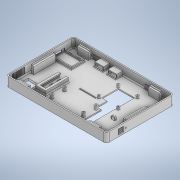
# Autodesk Inventor part: Bottom_new
Saved by Autodesk Inventor 2021 (Build 250183000, 183)
## iProperties
Created: 2020-06-14
Part Number: Bottom_new
Material: Generic
Document SubType Name: Modeling
Designer: Mariano
Density: 1 g/cm^3
Appearance: Default
Author: Mariano
Autodesk Inventor part; units mm, degrees
(part 1 of 3)
ref_plane "YZ Plane" through (0, 0, 0) normal (1, 0, 0) x (0, 1, 0)
ref_plane "XZ Plane" through (0, 0, 0) normal (0, 1, 0) x (-1, 0, 0)
sketch "Sketch1" plane through (0, 0, 0) normal (0, 1, 0) x (-1, 0, 0)
  line L0 (92.2, -62) -> (-92.2, -62)
  line L1 (-92.2, -62) -> (-92.2, 62)
  line L2 (-92.2, 62) -> (92.2, 62)
  line L3 (92.2, 62) -> (92.2, -62)
  line L4 (92.2, -62) -> (-92.2, 62) construction
  line L5 (-92.2, -62) -> (92.2, 62) construction
  point P0 (0, 0)
  dimension "d0" = 184.4
  dimension "d1" = 124
  constraints: 12 end point, 2 midpoint, 2 parallel, 1 horizontal, 1 perpendicular
  measures "d0" distance of L1.end L2.end
  measures "d1" distance of L2.end L0.start
extrude "Extrusion1" add sketch "Sketch1" along normal blind 17
fillet "Fillet1" radius 5 4 edges at (-92.2, 8.5, 62) (92.2, 8.5, 62) (92.2, 8.5, -62) (-92.2, 8.5, -62)
shell "Shell1" thickness 2 removed faces 1 at (29.0667, 17, 20.6667)
ref_plane "Work Plane4" through (0, 0, 20) normal (0, 0, 1) x (1, 0, 0)
sketch "Sketch28" plane through (0, 0, 20) normal (0, 0, 1) x (1, 0, 0)
  circle A0 centre (62.2, 4.5) radius 4
  line L0 (92.2, 17) -> (92.2, 0) projected
  circle A1 centre (62.2, 4.5) radius 2.5
  line L1 (58.2, 4.5) -> (58.2, 2)
  line L2 (87.2, 2) -> (-87.2, 2) construction
  line L3 (60.1894, 5.9858) -> (60.1894, 7.958)
  line L4 (64.2106, 5.9858) -> (64.2106, 7.958)
  line L5 (66.2, 4.5) -> (66.2, 2)
  point P0 (0, 0)
  point P1 (75.2, 2)
  dimension "d152" = 8
  dimension "d153" = 30
  dimension "d156" = 5
  dimension "d157" = 4.0211
  dimension "d158" = 1.9722
  constraints: 8 end point, 6 point on circle, 3 tangent, 2 centre point, 2 vertical, 1 coincident, 1 parallel, 1 perpendicular, 1 point on line
  measures "d152" diameter of A0
  measures "d153" distance from line of L0 A0.centre
  measures "d156" diameter of A1
  measures "d157" distance of L4.start L3.start
  measures "d158" distance of L4.start L4.end
extrude "Extrusion21" add sketch "Sketch28" against normal blind 3 contours A0 L3 A1 L4 picked at (65.6381, 3.986)
fillet "Fillet3" radius 10.5 2 edges at (60.1894, 5.9858, 18.5) (64.2106, 5.9858, 18.5)
ref_plane "Work Plane5" through (0, 16, 0) normal (0, 1, 0) x (1, 0, 0)
sketch "Sketch31" plane through (-87.2, 2, 60) normal (0, 1, 0) x (1, 0, 0)
  line L0 (2, 114.9) -> (172.4, 114.9) construction
  line L1 (172.4, 114.9) -> (172.4, 3) construction
  line L2 (172.4, 3) -> (2, 3) construction
  line L3 (2, 3) -> (2, 114.9) construction
  line L4 (87.2, 114.9) -> (87.2, 3) construction
  line L5 (2, 58.95) -> (172.4, 58.95) construction
  line L6 (12, 116.9) -> (32, 116.9)
  line L7 (32, 116.9) -> (32, 111.9)
  line L8 (32, 111.9) -> (12, 111.9)
  line L9 (12, 111.9) -> (12, 116.9)
  line L10 (0, 78.95) -> (5, 78.95)
  line L11 (5, 78.95) -> (5, 38.95)
  line L12 (4, 38.95) -> (0, 38.95)
  line L13 (0, 38.95) -> (0, 78.95)
  line L14 (174.4, 0) -> (0, 0) projected
  line L15 (0, 38.95) -> (5, 38.95)
  point P0 (87.2, 60)
  point P1 (32, 114.4)
  point P2 (5, 58.95)
  point P3 (2, 38.95)
  point P4 (4, 38.95)
  dimension "d188" = 170.4
  dimension "d189" = 111.9
  dimension "d190" = 20
  dimension "d191" = 5
  dimension "d192" = 10
  dimension "d198" = 40
  dimension "d199" = 5
  dimension "d256" = 3
  dimension "d389" = 3
  dimension "d502" = 2
  constraints: 30 end point, 7 midpoint, 7 parallel, 3 horizontal, 3 perpendicular, 3 point on line, 1 collinear
  measures "d188" distance of L0.start L0.end
  measures "d189" distance of L0.end L1.end
  measures "d190" distance of L7.end L8.end
  measures "d191" distance of L6.end L7.end
  measures "d192" distance between parallel lines of L3 L9
  measures "d198" distance of L10.end L11.end
  measures "d199" distance between parallel lines of L11 L13
  measures "d256" distance between parallel lines of L14 L2
  measures "d389" distance between parallel lines of L8 L0
  measures "d502" distance between parallel lines of L13 L3
extrude "Extrusion22" add sketch "Sketch31" along normal up to surface (14 mm away) contours L6 L7 L8 L9
sketch "Sketch32" plane through (-75.2, 16, -51.9) normal (0, 1, 0) x (1, 0, 0)
  line L0 (0, 0) -> (0, 6)
  line L1 (0, 3) -> (20, 3)
  line L2 (20, 6) -> (20, 0)
  line L3 (20, 0) -> (0, 0) projected
  line L4 (20, 0) -> (0, 0)
  line L5 (0, 0) -> (0, 3)
  point P0 (75.2, -51.9)
  dimension "d390" = 3
  constraints: 10 end point, 2 midpoint, 1 collinear, 1 perpendicular
  measures "d390" distance between parallel lines of L1 L3
extrude "Extrusion23" cut sketch "Sketch32" against normal blind 1.2
extrude "Extrusion24" add sketch "Sketch31" along normal up to surface (14 mm away) contours L10 L11 L15 L12 L13
sketch "Sketch33" plane through (-87.2, 16, 21.05) normal (0, 1, 0) x (1, 0, 0)
  line L0 (5, 40) -> (5, 0) projected
  line L1 (1.8, 0) -> (5, 0)
  line L2 (5, 0) -> (5, 40)
  line L3 (5, 40) -> (1.8, 40)
  line L4 (1.8, 40) -> (1.8, 0)
  line L5 (0, 0) -> (0, 40) projected
  point P0 (87.2, 21.05)
  dimension "d503" = 1.8
  constraints: 8 end point, 2 parallel, 1 horizontal, 1 perpendicular
  measures "d503" distance between parallel lines of L4 L5
extrude "Extrusion25" cut sketch "Sketch33" against normal blind 1.2
mirror "Mirror13" about plane through (0, 0, 0) normal (1, 0, 0) of "Extrusion24", "Extrusion25"
sketch "Sketch34" plane through (-87.2, 2, 60) normal (0, 1, 0) x (1, 0, 0)
  line L0 (103.971, 95) -> (134.4, 95)
  line L1 (134.4, 95) -> (134.4, 64.596)
  line L2 (134.4, 64.596) -> (103.971, 64.596)
  line L3 (103.971, 64.596) -> (103.971, 95)
  circle A0 centre (101.469, 97.502) radius 2.502
  line L4 (119.1855, 95) -> (119.1855, 64.596) construction
  line L5 (103.971, 79.798) -> (134.4, 79.798) construction
  circle A1 centre (136.902, 97.502) radius 2.502
  circle A2 centre (101.469, 62.094) radius 2.502
  circle A3 centre (136.902, 62.094) radius 2.502
  line L6 (0, 120) -> (174.4, 120) projected
  line L7 (177.4, 117) -> (177.4, 3) projected
  line L8 (109.4, 64.596) -> (134.4, 64.596)
  line L9 (134.4, 64.596) -> (134.4, 4.596)
  line L10 (134.4, 4.596) -> (122.4, 4.596)
  line L11 (122.4, 4.596) -> (122.4, 45.596)
  line L12 (122.4, 45.596) -> (114, 45.596)
  line L13 (114, 45.596) -> (114, 64.596)
  point P0 (87.2, 60)
  dimension "d204" = 30.429
  dimension "d205" = 30.404
  dimension "d206" = 5.004
  dimension "d207" = 2.502
  dimension "d208" = 2.502
  dimension "d209" = 25
  dimension "d210" = 43
  dimension "d227" = 12
  dimension "d228" = 60
  dimension "d387" = 20.4
  dimension "d388" = 41
  constraints: 24 end point, 4 centre point, 4 midpoint, 4 perpendicular, 3 parallel, 3 point on line, 3 symmetric about line, 2 horizontal, 1 vertical, 3 other
  measures "d204" distance of L1.end L2.end
  measures "d205" distance of L0.end L1.end
  measures "d206" diameter of A0
  measures "d207" distance from line of L3 A0.centre
  measures "d208" distance from line of L0 A0.centre
  measures "d209" distance between parallel lines of L0 L6
  measures "d210" distance between parallel lines of L7 L1
  measures "d227" distance of L9.end L10.end
  measures "d228" distance between parallel lines of L10 L2
  measures "d387" distance between parallel lines of L9 L13
  measures "d388" distance of L10.end L11.end
extrude "Extrusion27" add sketch "Sketch34" along normal blind 4 contours A3 | A0 | A1 | A2
extrude "Extrusion28" cut sketch "Sketch34" against normal through all contours L0 L1 L2 L3
extrude "Extrusion29" cut sketch "Sketch34" against normal through all contours L0 L1 L2 L3 | L9 L10 L11 L12 L13 L2
sketch "Sketch36" plane through (-87.2, 2, 60) normal (0, 1, 0) x (1, 0, 0)
  line L0 (22.24, 13) -> (7, 13)
  line L1 (7, 13) -> (7, 26.5)
  line L2 (7, 26.5) -> (22.24, 26.5)
  line L3 (22.24, 26.5) -> (22.24, 13)
  circle A0 centre (19.7, 11.26) radius 1.275
  line L4 (14.62, 13) -> (14.62, 26.5) construction
  circle A1 centre (9.54, 11.26) radius 1.275
  line L5 (0, 120) -> (174.4, 120) projected
  line L6 (-3, 3) -> (-3, 117) projected
  line L7 (-5, 117) -> (-5, 3) projected
  line L8 (0, -2) -> (174.4, -2) projected
  point P0 (87.2, 60)
  dimension "d231" = 15.24
  dimension "d232" = 13.5
  dimension "d233" = 2.55
  dimension "d234" = 15.24
  dimension "d235" = 2.54
  dimension "d511" = 12
  dimension "d512" = 15
  constraints: 10 end point, 2 centre point, 2 midpoint, 2 parallel, 1 perpendicular, 1 symmetric about line, 1 other
  measures "d231" distance of L1.end L2.end
  measures "d232" distance of L0.end L1.end
  measures "d233" diameter of A0
  measures "d234" distance from line of L2 A0.centre
  measures "d235" distance from line of L3 A0.centre
  measures "d511" distance between parallel lines of L7 L1
  measures "d512" distance between parallel lines of L8 L0
extrude "Extrusion30" add sketch "Sketch36" along normal blind 4 contours A0 | A1
extrude "Extrusion31" cut sketch "Sketch36" against normal through all contours L0 L1 L2 L3
sketch "Sketch35" plane through (-87.2, 2, 60) normal (0, 1, 0) x (1, 0, 0)
  line L0 (54.7, 45.5337) -> (119.7, 45.5337) construction
  line L1 (119.7, 45.5337) -> (119.7, 15.3337) construction
  line L2 (119.7, 15.3337) -> (54.7, 15.3337) construction
  line L3 (54.7, 15.3337) -> (54.7, 45.5337) construction
  circle A0 centre (58.2, 42.0337) radius 3
  line L4 (87.2, 45.5337) -> (87.2, 15.3337) construction
  line L5 (54.7, 30.4337) -> (119.7, 30.4337) construction
  circle A1 centre (116.2, 42.0337) radius 3
  circle A2 centre (58.2, 19.0337) radius 3
  line L6 (54.7, 15.3337) -> (119.7, 15.3337) construction
  circle A3 centre (116.2, 19.0337) radius 3
  point P0 (87.2, 60)
  dimension "d211" = 65
  dimension "d212" = 30.2
  dimension "d213" = 6
  dimension "d214" = 3.5
  dimension "d215" = 3.5
  dimension "d216" = 6
  dimension "d217" = 3.5
  dimension "d218" = 3.7
  constraints: 14 end point, 4 centre point, 4 midpoint, 4 symmetric about line, 2 parallel, 1 horizontal, 1 perpendicular, 1 point on line, 2 other
  measures "d211" distance of L1.end L2.end
  measures "d212" distance of L0.end L1.end
  measures "d213" diameter of A0
  measures "d214" distance from line of L0 A0.centre
  measures "d215" distance from line of L3 A0.centre
  measures "d216" diameter of A2
  measures "d217" distance from line of L3 A2.centre
  measures "d218" distance from line of L2 A2.centre
extrude "Extrusion26" add sketch "Sketch35" along normal blind 6
sketch "Sketch37" plane through (-29, 8, 40.9663) normal (0, 1, 0) x (1, 0, 0)
  circle A0 centre (0, 0) radius 3 projected
  circle A1 centre (0, 23) radius 3 projected
  circle A2 centre (58, 0) radius 3 projected
  circle A3 centre (58, 23) radius 3 projected
  point P0 (29, 40.9663)
  point P1 (0, 23)
  point P2 (58, 0)
  point P3 (58, 23)
  constraints: 4 coincident
hole "Hole10" at (-29, 8, 40.9663) at (-29, 8, 17.9663) at (29, 8, 40.9663) at (29, 8, 17.9663) direction (0, -1, 0) diameter 3 depth 6 tip angle 118
sketch "Sketch38" plane through (14.269, 6, -2.094) normal (0, 1, 0) x (1, 0, 0)
  circle A0 centre (0, 0) radius 2.502 projected
  circle A1 centre (0, 35.408) radius 2.502 projected
  circle A2 centre (35.433, 0) radius 2.502 projected
  arc A3 (37.935, 35.408) -> (37.935, 35.408) centre (35.433, 35.408) ccw projected
  point P0 (-14.269, -2.094)
  point P1 (0, 35.408)
  point P2 (35.433, 0)
  point P3 (35.433, 35.408)
  constraints: 4 coincident
hole "Hole11" at (14.269, 6, -2.094) at (14.269, 6, -37.502) at (49.702, 6, -2.094) at (49.702, 6, -37.502) direction (0, -1, 0) diameter 2 depth 4 tip angle 118
ref_plane "Work Plane8" through (-85.2, 2, 1.05) normal (0, 0, 1) x (1, 0, 0)
ref_plane "Work Plane9" through (0, 2, -54.9) normal (-1, 0, 0) x (0, 0, 1)
mirror "Mirror14" about plane through (0, 2, -54.9) normal (-1, 0, 0) of "Extrusion22", "Extrusion23"
mirror "Mirror15" about plane through (-85.2, 2, 1.05) normal (0, 0, 1) of "Extrusion22", "Extrusion23", "Mirror14"
sketch "Sketch40" plane through (-87.2, 2, -60) normal (0, 0, 1) x (1, 0, 0)
  line L0 (34, 7) -> (46, 7)
  line L1 (46, 7) -> (46, 5)
  line L2 (46, 5) -> (34, 5)
  line L3 (34, 5) -> (34, 7)
  line L4 (-5, 15) -> (0, 15) projected
  line L5 (0, 15) -> (0, -2) projected
  line L6 (0, -2) -> (-5, -2) projected
  line L7 (-5, -2) -> (-5, 15) projected
  line L8 (0, 15) -> (174.4, 15) projected
  point P0 (87.2, -2)
  dimension "d260" = 2
  dimension "d261" = 12
  dimension "d262" = 39
  dimension "d510" = 8
  constraints: 8 end point, 2 parallel, 1 horizontal, 1 perpendicular
  measures "d260" distance of L2.end L0.start
  measures "d261" distance of L1.end L2.end
  measures "d262" distance between parallel lines of L7 L3
  measures "d510" distance between parallel lines of L8 L0
extrude "Extrusion32" cut sketch "Sketch40" against normal blind 1.2 contours L0 L1 L2 L3
mirror "Mirror16" about plane through (0, 0, 0) normal (1, 0, 0) of "Extrusion32"
mirror "Mirror17" about plane through (0, 0, 0) normal (0, 0, 1) of "Extrusion32", "Mirror16"
sketch "Sketch44" plane through (-90.2, 2, -57) normal (1, 0, 0) x (0, 0, -1)
  line L0 (-63, 7) -> (-51, 7)
  line L1 (-51, 7) -> (-51, 5)
  line L2 (-51, 5) -> (-63, 5)
  line L3 (-63, 5) -> (-63, 7)
  line L4 (0, 15) -> (0, 0) projected
  line L5 (-114, 15) -> (0, 15) projected
  line L6 (-118, 15) -> (-114, 15) projected
  line L7 (-118, -2) -> (-118, 15) projected
  line L8 (4, -2) -> (-118, -2) projected
  line L9 (4, 15) -> (4, -2) projected
  line L10 (0, 15) -> (4, 15) projected
  line L11 (-114, 0) -> (0, 0) projected
  line L12 (-114, 15) -> (-114, 0) projected
  line L13 (0, 15) -> (0, 0) projected
  line L14 (-118, -2) -> (-118, 15) projected
  line L15 (4, -2) -> (-118, -2) projected
  line L16 (4, 15) -> (4, -2) projected
  line L17 (-114, 0) -> (0, 0) projected
  line L18 (-114, 15) -> (-114, 0) projected
  line L19 (-114, 15) -> (-119, 15) projected
  line L20 (-119, 15) -> (-119, -2) projected
  line L21 (-119, -2) -> (-114, -2) projected
  line L22 (-114, -2) -> (-114, 15) projected
  line L23 (-114, 0) -> (0, 0) projected
  line L24 (0, 15) -> (0, 0) projected
  line L25 (-118, -2) -> (-118, 15) projected
  line L26 (4, -2) -> (-118, -2) projected
  line L27 (4, 15) -> (4, -2) projected
  line L28 (-114, 15) -> (-114, 0) projected
  line L29 (29.8, -2) -> (-143.8, -2) projected
  line L30 (-57, -5.4) -> (-57, 18.4) projected
  line L31 (-114, 15) -> (0, 15) projected
  line L32 (-118, 15) -> (-114, 15) projected
  line L33 (0, 15) -> (4, 15) projected
  line L34 (-114, 15) -> (0, 15) projected
  line L35 (-118, 15) -> (-114, 15) projected
  line L36 (0, 15) -> (4, 15) projected
  point P0 (-57, -2)
  point P1 (-57, 5)
  dimension "d266" = 12
  dimension "d267" = 2
  dimension "d508" = 8
  constraints: 8 end point, 2 parallel, 1 horizontal, 1 midpoint, 1 perpendicular, 1 point on line
  measures "d266" distance of L1.end L2.end
  measures "d267" distance of L0.end L1.end
  measures "d508" distance between parallel lines of L5 L0
extrude "Extrusion33" cut sketch "Sketch44" against normal blind 1.2 contours L0 L30 L2 L3 | L0 L1 L2 L30
chamfer "Chamfer6" distance 2 angle 45 8 edges at (-90.2, 2, 0) (-89.3213, 2, -59.1213) (0, 2, -60) (89.3213, 2, -59.1213) (90.2, 2, 0) (-89.3213, 2, 59.1213) (0, 2, 60) (89.3213, 2, 59.1213)
ref_plane "Work Plane10" through (-87.2, 15.4, 21.05) normal (0, 1, 0) x (1, 0, 0)
sketch "Sketch50" plane through (-87.2, 15.4, 21.05) normal (0, 1, 0) x (1, 0, 0)
  line L0 (-3, 78.05) -> (-3, -35.95) projected
  line L1 (-1, -35.95) -> (-1, 78.05) projected
  line L2 (-3, 15.05) -> (-1, 15.05)
  line L3 (-1, 15.05) -> (-1, 27.05)
  line L4 (-1, 27.05) -> (-3, 27.05)
  line L5 (-3, 27.05) -> (-3, 15.05)
  point P0 (87.2, 21.05)
  point P1 (0, 17.975)
  point P2 (-3, -35.95)
  point P3 (2, 17.975)
  point P4 (2, -43)
  point P5 (2, -21.05)
  point P6 (-1, 78.05)
  point P7 (-1, 15.05)
  constraints: 8 end point, 2 parallel, 2 point on line, 1 horizontal, 1 perpendicular, 4 other
extrude "Extrusion40" cut sketch "Sketch50" against normal through all
sketch "Sketch53" plane through (87.2, 0, -62) normal (0, 0, -1) x (-1, 0, 0)
  line L0 (112.2, 7.7) -> (125.4, 7.7)
  line L1 (125.4, 7.7) -> (125.4, 2)
  line L2 (125.4, 2) -> (112.2, 2)
  line L3 (112.2, 2) -> (112.2, 7.7)
  line L4 (174.4, 2) -> (0, 2) projected
  line L5 (177.4, 4) -> (177.4, 17) projected
  line L6 (88.2, 2) -> (88.2, 7.7)
  line L7 (88.2, 7.7) -> (101.4, 7.7)
  line L8 (101.4, 7.7) -> (101.4, 2)
  line L9 (101.4, 2) -> (88.2, 2)
  point P0 (87.2, 0)
  point P1 (118.8, 2)
  point P2 (171.4, 4)
  point P3 (94.8, 2)
  point P4 (88.2, 2)
  point P5 (101.4, 2)
  dimension "d361" = 13.2
  dimension "d362" = 5.7
  dimension "d363" = 52
  dimension "d366" = 24
  constraints: 16 end point, 2 horizontal, 2 parallel, 1 midpoint, 1 perpendicular, 1 point on line, 10 other
  measures "d361" distance of L0.start L0.end
  measures "d362" distance of L0.end L1.end
  measures "d366" distance of L2.end L6.start
extrude "Extrusion45" cut sketch "Sketch53" against normal blind 4
sketch "Sketch57" plane through (87.2, 0, -62) normal (0, 0, -1) x (-1, 0, 0)
  line L0 (88.2, 7.7) -> (88.2, 4) projected
  line L1 (101.4, 2) -> (88.2, 2) projected
  line L2 (88.2, 7.7) -> (101.4, 7.7)
  line L3 (101.4, 7.7) -> (101.4, 2)
  line L4 (101.4, 2) -> (88.2, 2)
  line L5 (88.2, 2) -> (88.2, 7.7)
  line L6 (112.2, 7.7) -> (125.4, 7.7) projected
  line L7 (125.4, 2) -> (112.2, 2)
  line L8 (112.2, 2) -> (112.2, 7.7)
  line L9 (112.2, 7.7) -> (125.4, 7.7)
  line L10 (125.4, 7.7) -> (125.4, 2)
  line L11 (102.9, 9.2) -> (86.7, 9.2)
  line L12 (86.7, 9.2) -> (86.7, 0.5)
  line L13 (86.7, 0.5) -> (102.9, 0.5)
  line L14 (102.9, 0.5) -> (102.9, 9.2)
  line L15 (110.7, 9.2) -> (110.7, 0.5)
  line L16 (110.7, 0.5) -> (126.9, 0.5)
  line L17 (126.9, 0.5) -> (126.9, 9.2)
  line L18 (126.9, 9.2) -> (110.7, 9.2)
  point P0 (87.2, 0)
  dimension "d379" = 1.5
  dimension "d380" = 1.5
  constraints: 32 end point, 8 parallel, 4 perpendicular, 2 horizontal, 6 other
  measures "d379" distance between parallel lines of L2 L11
  measures "d380" distance between parallel lines of L8 L15
extrude "Extrusion46" add sketch "Sketch57" against normal blind 13.2
sketch "Sketch58" plane through (87.2, 0, -62) normal (0, 0, -1) x (-1, 0, 0)
  line L0 (88.2, 7.7) -> (101.4, 7.7) projected
  line L1 (88.2, 7.7) -> (101.4, 7.7)
  line L2 (101.4, 7.7) -> (101.4, 2)
  line L3 (101.4, 2) -> (88.2, 2)
  line L4 (88.2, 2) -> (88.2, 7.7)
  line L5 (112.2, 7.7) -> (125.4, 7.7) projected
  line L6 (125.4, 2) -> (125.4, 7.7) projected
  line L7 (112.2, 7.7) -> (125.4, 7.7)
  line L8 (125.4, 7.7) -> (125.4, 2)
  line L9 (125.4, 2) -> (112.2, 2)
  line L10 (112.2, 2) -> (112.2, 7.7)
  line L11 (87.6, 8.3) -> (102, 8.3)
  line L12 (102, 8.3) -> (102, 1.4)
  line L13 (102, 1.4) -> (87.6, 1.4)
  line L14 (87.6, 1.4) -> (87.6, 8.3)
  line L15 (111.6, 8.3) -> (126, 8.3)
  line L16 (126, 8.3) -> (126, 1.4)
  line L17 (126, 1.4) -> (111.6, 1.4)
  line L18 (111.6, 1.4) -> (111.6, 8.3)
  point P0 (87.2, 0)
  dimension "d383" = 0.6
  dimension "d384" = 0.6
  constraints: 32 end point, 8 parallel, 4 perpendicular, 2 horizontal, 6 other
  measures "d383" distance between parallel lines of L4 L14
  measures "d384" distance between parallel lines of L10 L18
extrude "Extrusion47" cut sketch "Sketch58" against normal blind 0.5
chamfer "Chamfer7" distance 2 angle 45 3 edges at (-64.96, 2, 40.25) (-72.58, 2, 33.5) (-80.2, 2, 40.25)
sketch "Sketch60" plane through (0, 0, 0) normal (0, -1, 0) x (1, 0, 0)
  line L0 (87.2, -60) -> (0.5, -60) projected
  line L1 (53.2, -60) -> (41.2, -60)
  line L2 (41.2, -60) -> (41.2, -58)
  line L3 (41.2, -58) -> (53.2, -58)
  line L4 (53.2, -58) -> (53.2, -60)
  point P0 (0, 0)
  dimension "d395" = 2
  constraints: 8 end point, 2 parallel, 1 horizontal, 1 perpendicular
  measures "d395" distance of L1.end L2.end
extrude "Extrusion48" cut sketch "Sketch60" against normal through all
mirror "Mirror22" about plane through (0, 0, 0) normal (1, 0, 0) of "Extrusion48"
mirror "Mirror23" about plane through (0, 0, 0) normal (0, 0, 1) of "Extrusion48", "Mirror22"
sketch "Sketch61" plane through (-75.2, 2, 54) normal (0, 1, 0) x (1, 0, 0)
  line L0 (-16, 77.3) -> (17.3, 77.3)
  line L1 (17.3, 77.3) -> (17.3, 98)
  line L2 (17.3, 98) -> (-16, 98)
  line L3 (-16, 98) -> (-16, 77.3)
  line L4 (-17, 111) -> (-17, -3) projected
  line L5 (162.4, 116) -> (-12, 116) projected
  line L6 (-16, 78.3) -> (17.3, 78.3)
  line L7 (17.3, 97) -> (-16, 97)
  point P0 (75.2, 54)
  dimension "d398" = 33.3
  dimension "d399" = 1
  dimension "d400" = 18
  dimension "d401" = 20.7
  dimension "d414" = 1
  dimension "d415" = 1
  constraints: 12 end point, 4 point on line, 3 perpendicular, 2 parallel, 1 horizontal
  measures "d398" distance of L1.end L2.end
  measures "d399" distance between parallel lines of L4 L3
  measures "d400" distance between parallel lines of L5 L2
  measures "d401" distance of L0.end L1.end
  measures "d414" distance between parallel lines of L6 L0
  measures "d415" distance between parallel lines of L7 L2
sketch "Sketch62" plane through (-90.2, 17, 57) normal (1, 0, 0) x (0, 0, -1)
  line L0 (51, -8) -> (63, -8) projected
  line L1 (51, -13) -> (51, -17) projected
  line L2 (63, -17) -> (51, -17) projected
  line L3 (118, -17) -> (63, -17) projected
  line L4 (118, 0) -> (118, -17) projected
  line L5 (114, 0) -> (118, 0) projected
  line L6 (114, 0) -> (114, -13) projected
  line L7 (63, -13) -> (114, -13) projected
  line L8 (63, -17) -> (63, -13) projected
  line L9 (0, -13) -> (51, -13) projected
  line L10 (0, 0) -> (0, -13) projected
  line L11 (0, 0) -> (114, 0) projected
  line L12 (51, -17) -> (-4, -17) projected
  line L13 (-4, -17) -> (-4, 0) projected
  line L14 (-4, 0) -> (0, 0) projected
  line L15 (63, -10) -> (63, -8) projected
  line L16 (63, -8) -> (51, -8) projected
  line L17 (51, -8) -> (51, -10) projected
  line L18 (51, -10) -> (63, -10) projected
  line L19 (101, -13.5) -> (80.3, -13.5)
  line L20 (80.3, -13.5) -> (80.3, -8.5)
  line L21 (80.3, -8.5) -> (101, -8.5)
  line L22 (101, -8.5) -> (101, -13.5)
  line L23 (51, -13) -> (51, -17) projected
  line L24 (63, -17) -> (51, -17) projected
  line L25 (118, -17) -> (63, -17) projected
  line L26 (118, 0) -> (118, -17) projected
  line L27 (114, 0) -> (118, 0) projected
  line L28 (114, 0) -> (114, -13) projected
  line L29 (63, -13) -> (114, -13) projected
  line L30 (63, -17) -> (63, -13) projected
  line L31 (0, -13) -> (51, -13) projected
  line L32 (0, 0) -> (0, -13) projected
  line L33 (0, 0) -> (114, 0) projected
  line L34 (51, -17) -> (-4, -17) projected
  line L35 (-4, -17) -> (-4, 0) projected
  line L36 (-4, 0) -> (0, 0) projected
  line L37 (63, -10) -> (63, -8) projected
  line L38 (63, -8) -> (51, -8) projected
  line L39 (51, -8) -> (51, -10) projected
  line L40 (51, -13) -> (51, -17) projected
  line L41 (63, -17) -> (51, -17) projected
  line L42 (118, -17) -> (63, -17) projected
  line L43 (118, 0) -> (118, -17) projected
  line L44 (114, 0) -> (118, 0) projected
  line L45 (114, 0) -> (114, -13) projected
  line L46 (63, -13) -> (114, -13) projected
  line L47 (63, -17) -> (63, -13) projected
  line L48 (0, -13) -> (51, -13) projected
  line L49 (0, 0) -> (0, -13) projected
  line L50 (0, 0) -> (114, 0) projected
  line L51 (51, -17) -> (-4, -17) projected
  line L52 (-4, -17) -> (-4, 0) projected
  line L53 (-4, 0) -> (0, 0) projected
  line L54 (63, -10) -> (63, -8) projected
  line L55 (63, -8) -> (51, -8) projected
  line L56 (51, -8) -> (51, -10) projected
  line L57 (51, -13) -> (51, -17) projected
  line L58 (63, -17) -> (51, -17) projected
  line L59 (118, -17) -> (63, -17) projected
  line L60 (118, 0) -> (118, -17) projected
  line L61 (114, 0) -> (118, 0) projected
  line L62 (114, 0) -> (114, -13) projected
  line L63 (63, -13) -> (114, -13) projected
  line L64 (63, -17) -> (63, -13) projected
  line L65 (0, -13) -> (51, -13) projected
  line L66 (0, 0) -> (0, -13) projected
  line L67 (0, 0) -> (114, 0) projected
  line L68 (51, -17) -> (-4, -17) projected
  line L69 (-4, -17) -> (-4, 0) projected
  line L70 (-4, 0) -> (0, 0) projected
  line L71 (63, -10) -> (63, -8) projected
  line L72 (63, -8) -> (51, -8) projected
  line L73 (51, -8) -> (51, -10) projected
  line L74 (101, -15) -> (80.3, -15) projected
  line L75 (51, -10) -> (63, -10) projected
  line L76 (51, -10) -> (63, -10) projected
  line L77 (51, -10) -> (63, -10) projected
  point P0 (57, -17)
  point P1 (101, -15)
  point P2 (101, -15)
  dimension "d403" = 5
  dimension "d411" = 1.5
  constraints: 8 end point, 2 parallel, 2 point on line, 1 horizontal, 1 perpendicular
  measures "d403" distance of L21.end L19.start
  measures "d411" distance between parallel lines of L19 L74
extrude "Extrusion49" cut sketch "Sketch62" against normal blind 1 contours L20 L21 L22 L7 | L7 L22 L19 L20
sketch "Sketch63" plane through (-91.2, 17, 57) normal (1, 0, 0) x (0, 0, -1)
  line L0 (84.3, -7) -> (96, -7)
  line L1 (96, -7) -> (96, -13.5)
  line L2 (96, -13.5) -> (84.3, -13.5)
  line L3 (84.3, -13.5) -> (84.3, -7)
  line L4 (80.3, -8.5) -> (80.3, -13.5) projected
  line L5 (80.3, -13.5) -> (101, -13.5) projected
  line L6 (101, -13.5) -> (101, -8.5) projected
  line L7 (101, -8.5) -> (80.3, -8.5) projected
  line L8 (117, -17) -> (-3, -17) projected
  line L9 (-3, -17) -> (-3, 0) projected
  line L10 (-3, 0) -> (117, 0) projected
  line L11 (117, 0) -> (117, -17) projected
  line L12 (63, -10) -> (63, -8) projected
  line L13 (63, -8) -> (51, -8) projected
  line L14 (51, -8) -> (51, -10) projected
  line L15 (51, -10) -> (63, -10) projected
  point P0 (57, -17)
  point P1 (90.65, -13.5)
  point P2 (96, -8.5)
  point P3 (84.3, -8.5)
  dimension "d406" = 4
  dimension "d407" = 5
  dimension "d408" = 6.5
  constraints: 8 end point, 2 parallel, 1 horizontal, 1 midpoint, 1 perpendicular, 1 point on line
  measures "d406" distance between parallel lines of L4 L3
  measures "d407" distance between parallel lines of L6 L1
  measures "d408" distance of L0.end L1.end
sketch "Sketch64" plane through (-75.2, 2, 54) normal (0, 1, 0) x (1, 0, 0)
  line L0 (12.24, 7) -> (12.24, 22.5) projected
  line L1 (12.24, 22.5) -> (-7, 22.5) projected
  line L2 (-7, 22.5) -> (-7, 7) projected
  line L3 (-7, 7) -> (12.24, 7) projected
  line L4 (150.4, 110.9) -> (150.4, 105.9) projected
  line L5 (150.4, 105.9) -> (130.4, 105.9) projected
  line L6 (130.4, 105.9) -> (130.4, 110.9) projected
  line L7 (130.4, 110.9) -> (150.4, 110.9) projected
  circle A0 centre (124.902, 56.094) radius 1 projected
  circle A1 centre (89.469, 56.094) radius 1 projected
  circle A2 centre (89.469, 91.502) radius 1 projected
  circle A3 centre (124.902, 91.502) radius 1 projected
  circle A4 centre (104.2, 13.0337) radius 1.5 projected
  circle A5 centre (46.2, 13.0337) radius 1.5 projected
  circle A6 centre (46.2, 36.0337) radius 1.5 projected
  circle A7 centre (104.2, 36.0337) radius 1.5 projected
  circle A8 centre (104.2, 13.0337) radius 3 projected
  circle A9 centre (46.2, 13.0337) radius 3 projected
  circle A10 centre (104.2, 36.0337) radius 3 projected
  circle A11 centre (46.2, 36.0337) radius 3 projected
  circle A12 centre (-2.46, 5.26) radius 1.275 projected
  circle A13 centre (7.7, 5.26) radius 1.275 projected
  line L8 (91.971, 89) -> (91.971, 58.596) projected
  line L9 (91.971, 58.596) -> (102, 58.596) projected
  line L10 (102, 58.596) -> (102, 39.596) projected
  line L11 (102, 39.596) -> (110.4, 39.596) projected
  line L12 (110.4, 39.596) -> (110.4, -1.404) projected
  line L13 (110.4, -1.404) -> (122.4, -1.404) projected
  line L14 (122.4, -1.404) -> (122.4, 56.094) projected
  circle A14 centre (124.902, 56.094) radius 2.502 projected
  line L15 (122.4, 56.094) -> (122.4, 89) projected
  line L16 (122.4, 89) -> (91.971, 89) projected
  circle A15 centre (89.469, 56.094) radius 2.502 projected
  circle A16 centre (124.902, 91.502) radius 2.502 projected
  circle A17 centre (89.469, 91.502) radius 2.502 projected
  line L17 (157.4, 72.95) -> (162.4, 72.95) projected
  line L18 (162.4, 72.95) -> (162.4, 32.95) projected
  line L19 (157.4, 32.95) -> (157.4, 72.95) projected
  line L20 (-7, 72.95) -> (-7, 32.95) projected
  line L21 (-12, 32.95) -> (-12, 72.95) projected
  line L22 (-12, 72.95) -> (-7, 72.95) projected
  line L23 (20, 110.9) -> (20, 105.9) projected
  line L24 (20, 105.9) -> (0, 105.9) projected
  line L25 (0, 105.9) -> (0, 110.9) projected
  line L26 (0, 110.9) -> (20, 110.9) projected
  line L27 (137.4, 37) -> (137.4, 34) projected
  line L28 (137.4, 34) -> (134.2775, 34) projected
  line L29 (134.2775, 34) -> (134.2775, 37) projected
  line L30 (134.2775, 37) -> (137.4, 37) projected
  line L31 (137.4, 37) -> (140.5225, 37) projected
  line L32 (140.5225, 37) -> (140.5225, 34) projected
  line L33 (140.5225, 34) -> (137.4, 34) projected
  arc A18 (-12, 116) -> (-17, 111) centre (-12, 111) ccw projected
  line L34 (-12, 116) -> (36.4, 116) projected
  line L35 (36.4, 116) -> (36.4, 115.5) projected
  line L36 (36.4, 115.5) -> (37, 115.5) projected
  line L37 (37, 115.5) -> (50.2, 115.5) projected
  line L38 (50.2, 115.5) -> (50.8, 115.5) projected
  line L39 (50.8, 115.5) -> (50.8, 116) projected
  line L40 (50.8, 116) -> (60.4, 116) projected
  line L41 (60.4, 116) -> (60.4, 115.5) projected
  line L42 (60.4, 115.5) -> (61, 115.5) projected
  line L43 (61, 115.5) -> (74.2, 115.5) projected
  line L44 (74.2, 115.5) -> (74.8, 115.5) projected
  line L45 (74.8, 115.5) -> (74.8, 116) projected
  line L46 (74.8, 116) -> (162.4, 116) projected
  arc A19 (167.4, 111) -> (162.4, 116) centre (162.4, 111) ccw projected
  line L47 (167.4, 111) -> (167.4, -3) projected
  arc A20 (162.4, -8) -> (167.4, -3) centre (162.4, -3) ccw projected
  line L48 (162.4, -8) -> (-12, -8) projected
  arc A21 (-17, -3) -> (-12, -8) centre (-12, -3) ccw projected
  line L49 (-17, -3) -> (-17, 111) projected
  line L50 (37, 115.5) -> (37, 102.8) projected
  line L51 (37, 102.8) -> (35.5, 102.8) projected
  line L52 (35.5, 102.8) -> (35.5, 112) projected
  line L53 (35.5, 112) -> (34, 112) projected
  line L54 (34, 112) -> (34, 114) projected
  line L55 (34, 114) -> (22, 114) projected
  line L56 (22, 114) -> (22, 112) projected
  line L57 (22, 112) -> (-12, 112) projected
  arc A22 (-12, 112) -> (-13, 111) centre (-12, 111) ccw projected
  line L58 (-13, 111) -> (-13, 60) projected
  line L59 (-13, 48) -> (-13, 60) projected
  line L60 (-15, 48) -> (-13, 48) projected
  line L61 (-15, 60) -> (-15, 48) projected
  line L62 (-13, 60) -> (-15, 60) projected
  line L63 (50.2, 102.8) -> (50.2, 115.5) projected
  line L64 (51.7, 102.8) -> (50.2, 102.8) projected
  line L65 (51.7, 112) -> (51.7, 102.8) projected
  line L66 (59.5, 112) -> (51.7, 112) projected
  line L67 (59.5, 102.8) -> (59.5, 112) projected
  line L68 (61, 102.8) -> (59.5, 102.8) projected
  line L69 (61, 115.5) -> (61, 102.8) projected
  line L70 (74.2, 102.8) -> (74.2, 115.5) projected
  line L71 (75.7, 102.8) -> (74.2, 102.8) projected
  line L72 (75.7, 112) -> (75.7, 102.8) projected
  line L73 (116.4, 112) -> (75.7, 112) projected
  line L74 (116.4, 112) -> (128.4, 112) projected
  line L75 (162.4, 112) -> (128.4, 112) projected
  arc A23 (163.4, 111) -> (162.4, 112) centre (162.4, 111) ccw projected
  line L76 (163.4, -3) -> (163.4, 111) projected
  arc A24 (162.4, -4) -> (163.4, -3) centre (162.4, -3) ccw projected
  line L77 (150.4, -4) -> (162.4, -4) projected
  line L78 (150.4, 0) -> (150.4, -4) projected
  line L79 (130.4, 0) -> (150.4, 0) projected
  line L80 (130.4, -4) -> (130.4, 0) projected
  line L81 (128.4, -4) -> (130.4, -4) projected
  line L82 (128.4, -4) -> (116.4, -4) projected
  line L83 (34, -4) -> (116.4, -4) projected
  line L84 (34, -4) -> (22, -4) projected
  line L85 (20, -4) -> (22, -4) projected
  line L86 (20, 0) -> (20, -4) projected
  line L87 (0, 0) -> (20, 0) projected
  line L88 (0, -4) -> (0, 0) projected
  line L89 (-12, -4) -> (0, -4) projected
  arc A25 (-13, -3) -> (-12, -4) centre (-12, -3) ccw projected
  line L90 (-13, 48) -> (-13, -3) projected
  line L91 (22, 112) -> (34, 112) projected
  line L92 (116.4, 114) -> (116.4, 112) projected
  line L93 (128.4, 114) -> (116.4, 114) projected
  line L94 (128.4, 112) -> (128.4, 114) projected
  line L95 (128.4, -6) -> (128.4, -4) projected
  line L96 (116.4, -6) -> (128.4, -6) projected
  line L97 (116.4, -4) -> (116.4, -6) projected
  line L98 (34, -6) -> (34, -4) projected
  line L99 (22, -6) -> (34, -6) projected
  line L100 (22, -4) -> (22, -6) projected
  line L101 (150.4, 110.9) -> (150.4, 105.9) projected
  line L102 (150.4, 105.9) -> (130.4, 105.9) projected
  line L103 (130.4, 105.9) -> (130.4, 110.9) projected
  line L104 (130.4, 110.9) -> (150.4, 110.9) projected
  circle A26 centre (124.902, 56.094) radius 1 projected
  circle A27 centre (89.469, 56.094) radius 1 projected
  circle A28 centre (89.469, 91.502) radius 1 projected
  circle A29 centre (124.902, 91.502) radius 1 projected
  circle A30 centre (104.2, 13.0337) radius 1.5 projected
  circle A31 centre (46.2, 13.0337) radius 1.5 projected
  circle A32 centre (46.2, 36.0337) radius 1.5 projected
  circle A33 centre (104.2, 36.0337) radius 1.5 projected
  circle A34 centre (104.2, 13.0337) radius 3 projected
  circle A35 centre (46.2, 13.0337) radius 3 projected
  circle A36 centre (104.2, 36.0337) radius 3 projected
  circle A37 centre (46.2, 36.0337) radius 3 projected
  circle A38 centre (-2.46, 5.26) radius 1.275 projected
  circle A39 centre (7.7, 5.26) radius 1.275 projected
  line L105 (91.971, 89) -> (91.971, 58.596) projected
  line L106 (91.971, 58.596) -> (102, 58.596) projected
  line L107 (102, 58.596) -> (102, 39.596) projected
  line L108 (102, 39.596) -> (110.4, 39.596) projected
  line L109 (110.4, 39.596) -> (110.4, -1.404) projected
  line L110 (110.4, -1.404) -> (122.4, -1.404) projected
  line L111 (122.4, -1.404) -> (122.4, 56.094) projected
  circle A40 centre (124.902, 56.094) radius 2.502 projected
  line L112 (122.4, 56.094) -> (122.4, 89) projected
  line L113 (122.4, 89) -> (91.971, 89) projected
  circle A41 centre (89.469, 56.094) radius 2.502 projected
  circle A42 centre (124.902, 91.502) radius 2.502 projected
  circle A43 centre (89.469, 91.502) radius 2.502 projected
  line L114 (157.4, 72.95) -> (162.4, 72.95) projected
  line L115 (162.4, 72.95) -> (162.4, 32.95) projected
  line L116 (-12, 32.95) -> (-12, 72.95) projected
  line L117 (-12, 72.95) -> (-7, 72.95) projected
  line L118 (20, 110.9) -> (20, 105.9) projected
  line L119 (20, 105.9) -> (0, 105.9) projected
  line L120 (0, 105.9) -> (0, 110.9) projected
  line L121 (0, 110.9) -> (20, 110.9) projected
  arc A44 (-12, 116) -> (-17, 111) centre (-12, 111) ccw projected
  line L122 (-12, 116) -> (36.4, 116) projected
  line L123 (36.4, 116) -> (36.4, 115.5) projected
  line L124 (36.4, 115.5) -> (37, 115.5) projected
  line L125 (37, 115.5) -> (50.2, 115.5) projected
  line L126 (50.8, 116) -> (60.4, 116) projected
  line L127 (60.4, 116) -> (60.4, 115.5) projected
  line L128 (60.4, 115.5) -> (61, 115.5) projected
  line L129 (61, 115.5) -> (74.2, 115.5) projected
  line L130 (74.8, 116) -> (162.4, 116) projected
  arc A45 (167.4, 111) -> (162.4, 116) centre (162.4, 111) ccw projected
  line L131 (167.4, 111) -> (167.4, -3) projected
  arc A46 (162.4, -8) -> (167.4, -3) centre (162.4, -3) ccw projected
  line L132 (162.4, -8) -> (-12, -8) projected
  arc A47 (-17, -3) -> (-12, -8) centre (-12, -3) ccw projected
  line L133 (-17, -3) -> (-17, 111) projected
  line L134 (37, 115.5) -> (37, 102.8) projected
  line L135 (37, 102.8) -> (35.5, 102.8) projected
  line L136 (35.5, 102.8) -> (35.5, 112) projected
  line L137 (35.5, 112) -> (34, 112) projected
  line L138 (34, 112) -> (34, 114) projected
  line L139 (34, 114) -> (22, 114) projected
  line L140 (22, 114) -> (22, 112) projected
  line L141 (22, 112) -> (-12, 112) projected
  arc A48 (-12, 112) -> (-13, 111) centre (-12, 111) ccw projected
  line L142 (-13, 111) -> (-13, 60) projected
  line L143 (-13, 48) -> (-13, 60) projected
  line L144 (-15, 48) -> (-13, 48) projected
  line L145 (-15, 60) -> (-15, 48) projected
  line L146 (-13, 60) -> (-15, 60) projected
  line L147 (59.5, 112) -> (51.7, 112) projected
  line L148 (59.5, 102.8) -> (59.5, 112) projected
  line L149 (61, 102.8) -> (59.5, 102.8) projected
  line L150 (61, 115.5) -> (61, 102.8) projected
  line L151 (116.4, 112) -> (75.7, 112) projected
  line L152 (116.4, 112) -> (128.4, 112) projected
  line L153 (162.4, 112) -> (128.4, 112) projected
  arc A49 (163.4, 111) -> (162.4, 112) centre (162.4, 111) ccw projected
  line L154 (163.4, -3) -> (163.4, 111) projected
  arc A50 (162.4, -4) -> (163.4, -3) centre (162.4, -3) ccw projected
  line L155 (150.4, -4) -> (162.4, -4) projected
  line L156 (150.4, 0) -> (150.4, -4) projected
  line L157 (130.4, 0) -> (150.4, 0) projected
  line L158 (130.4, -4) -> (130.4, 0) projected
  line L159 (128.4, -4) -> (130.4, -4) projected
  line L160 (128.4, -4) -> (116.4, -4) projected
  line L161 (34, -4) -> (116.4, -4) projected
  line L162 (34, -4) -> (22, -4) projected
  line L163 (20, -4) -> (22, -4) projected
  line L164 (20, 0) -> (20, -4) projected
  line L165 (0, 0) -> (20, 0) projected
  line L166 (0, -4) -> (0, 0) projected
  line L167 (-12, -4) -> (0, -4) projected
  arc A51 (-13, -3) -> (-12, -4) centre (-12, -3) ccw projected
  line L168 (-13, 48) -> (-13, -3) projected
  line L169 (22, 112) -> (34, 112) projected
  line L170 (116.4, 114) -> (116.4, 112) projected
  line L171 (128.4, 114) -> (116.4, 114) projected
  line L172 (128.4, 112) -> (128.4, 114) projected
  line L173 (128.4, -6) -> (128.4, -4) projected
  line L174 (116.4, -6) -> (128.4, -6) projected
  line L175 (116.4, -4) -> (116.4, -6) projected
  line L176 (34, -6) -> (34, -4) projected
  line L177 (22, -6) -> (34, -6) projected
  line L178 (22, -4) -> (22, -6) projected
  line L179 (-15, -3) -> (-15, 111) projected
  line L180 (-16, 77.3) -> (17.3, 77.3) projected
  line L181 (17.3, 98) -> (-16, 98) projected
  line L182 (-13, 77.3) -> (-15, 77.3)
  line L183 (-15, 77.3) -> (-15, 98)
  line L184 (-15, 98) -> (-13, 98)
  line L185 (-13, 98) -> (-13, 77.3)
  line L186 (137.4, 37) -> (137.4, 34) projected
  line L187 (137.4, 34) -> (134.2775, 34) projected
  line L188 (134.2775, 34) -> (134.2775, 37) projected
  line L189 (134.2775, 37) -> (137.4, 37) projected
  line L190 (137.4, 37) -> (140.5225, 37) projected
  line L191 (140.5225, 37) -> (140.5225, 34) projected
  line L192 (140.5225, 34) -> (137.4, 34) projected
  line L193 (12.24, 7) -> (12.24, 22.5) projected
  line L194 (12.24, 22.5) -> (-7, 22.5) projected
  line L195 (-7, 22.5) -> (-7, 7) projected
  line L196 (-7, 7) -> (12.24, 7) projected
  line L197 (50.2, 115.5) -> (50.8, 115.5) projected
  line L198 (50.8, 115.5) -> (50.8, 116) projected
  line L199 (74.2, 115.5) -> (74.8, 115.5) projected
  line L200 (74.8, 115.5) -> (74.8, 116) projected
  line L201 (50.2, 102.8) -> (50.2, 115.5) projected
  line L202 (51.7, 102.8) -> (50.2, 102.8) projected
  line L203 (51.7, 112) -> (51.7, 102.8) projected
  line L204 (74.2, 102.8) -> (74.2, 115.5) projected
  line L205 (75.7, 102.8) -> (74.2, 102.8) projected
  line L206 (75.7, 112) -> (75.7, 102.8) projected
  line L207 (162.4, 32.95) -> (157.4, 32.95) projected
  line L208 (157.4, 32.95) -> (157.4, 72.95) projected
  line L209 (-7, 72.95) -> (-7, 32.95) projected
  line L210 (-7, 32.95) -> (-12, 32.95) projected
  line L211 (162.4, 32.95) -> (157.4, 32.95) projected
  line L212 (-7, 32.95) -> (-12, 32.95) projected
  point P0 (75.2, 54)
  point P1 (-13, 98)
  point P2 (6.9482, 0)
  constraints: 8 end point, 4 point on line, 2 horizontal alignment, 2 parallel, 1 horizontal, 1 perpendicular
extrude "Extrusion51" cut sketch "Sketch64" against normal up to surface contours L58 L180 L179 L181 surface through (-89.2, 3, -31) normal (0.7071068, 0.7071068, 0)
extrude "Extrusion52" add sketch "Sketch61" along normal blind 1.5 contours L3 L6 L1 L0 | L3 L2 L1 L7
sketch "Sketch65" plane through (-75.2, 2, 54) normal (0, 1, 0) x (1, 0, 0)
  line L0 (34, -4) -> (22, -4) projected
  line L1 (22, -4) -> (22, -6) projected
  line L2 (22, -6) -> (34, -6) projected
  line L3 (34, -6) -> (34, -4) projected
  line L4 (128.4, -4) -> (116.4, -4) projected
  line L5 (116.4, -4) -> (116.4, -6) projected
  line L6 (116.4, -6) -> (128.4, -6) projected
  line L7 (128.4, -6) -> (128.4, -4) projected
  line L8 (22, 112) -> (34, 112) projected
  line L9 (34, 112) -> (34, 114) projected
  line L10 (34, 114) -> (22, 114) projected
  line L11 (22, 114) -> (22, 112) projected
  line L12 (128.4, 114) -> (116.4, 114) projected
  line L13 (116.4, 114) -> (116.4, 112) projected
  line L14 (116.4, 112) -> (128.4, 112) projected
  line L15 (128.4, 112) -> (128.4, 114) projected
  line L16 (-15, 48) -> (-13, 48) projected
  line L17 (-13, 48) -> (-13, 60) projected
  line L18 (-13, 60) -> (-15, 60) projected
  line L19 (-15, 60) -> (-15, 48) projected
  line L20 (-5, 7) -> (10.24, 7) projected
  line L21 (10.24, 20.5) -> (-5, 20.5) projected
  arc A0 (-12, 116) -> (-17, 111) centre (-12, 111) ccw projected
  line L22 (162.4, 116) -> (-12, 116) projected
  arc A1 (167.4, 111) -> (162.4, 116) centre (162.4, 111) ccw projected
  line L23 (167.4, -3) -> (167.4, 111) projected
  arc A2 (162.4, -8) -> (167.4, -3) centre (162.4, -3) ccw projected
  line L24 (-12, -8) -> (162.4, -8) projected
  arc A3 (-17, -3) -> (-12, -8) centre (-12, -3) ccw projected
  line L25 (-17, 111) -> (-17, -3) projected
  line L26 (102, 58.596) -> (102, 39.596) projected
  line L27 (102, 39.596) -> (110.4, 39.596) projected
  line L28 (110.4, 39.596) -> (110.4, -1.404) projected
  line L29 (110.4, -1.404) -> (122.4, -1.404) projected
  line L30 (122.4, -1.404) -> (122.4, 89) projected
  line L31 (122.4, 89) -> (91.971, 89) projected
  line L32 (91.971, 89) -> (91.971, 58.596) projected
  line L33 (91.971, 58.596) -> (102, 58.596) projected
  line L34 (-14.5, 77.3) -> (17.3, 77.3) projected
  line L35 (17.3, 98) -> (-14.5, 98) projected
  line L36 (17.3, 77.3) -> (17.3, 78.3) projected
  line L37 (17.3, 97) -> (17.3, 98) projected
  line L38 (-13, 60) -> (-13, 77.3) projected
  line L39 (-13, 98) -> (-13, 111) projected
  line L40 (-13, 77.3) -> (19.3, 77.3)
  line L41 (19.3, 77.3) -> (19.3, 75.3)
  line L42 (19.3, 75.3) -> (-13, 75.3)
  line L43 (-13, 75.3) -> (-13, 77.3)
  line L44 (17.3, 77.3) -> (19.3, 77.3)
  line L45 (19.3, 77.3) -> (19.3, 98)
  line L46 (19.3, 98) -> (17.3, 98)
  line L47 (17.3, 98) -> (17.3, 77.3)
  line L48 (-13, 98) -> (19.3, 98)
  line L49 (19.3, 98) -> (19.3, 100)
  line L50 (19.3, 100) -> (-13, 100)
  line L51 (-13, 100) -> (-13, 98)
  line L52 (-5, 20.5) -> (-5, 7) projected
  line L53 (10.24, 7) -> (10.24, 20.5) projected
  point P0 (75.2, 54)
  point P1 (19.3, 98)
  point P2 (-13, 100)
  dimension "d418" = 2
  dimension "d419" = 2
  dimension "d420" = 2
  constraints: 24 end point, 6 parallel, 3 horizontal, 3 perpendicular, 2 point on line
  measures "d418" distance between parallel lines of L42 L34
  measures "d419" distance between parallel lines of L45 L47
  measures "d420" distance between parallel lines of L50 L48
extrude "Extrusion53" cut sketch "Sketch63" against normal through all contours L0 L1 L7 L3 | L7 L1 L2 L3
extrude "Extrusion54" add sketch "Sketch65" along normal blind 4.2 contours L34 L40 L41 L42 L38 | L46 L35 L39 L50 L49
sketch "Sketch66" plane through (-75.2, 2, 54) normal (0, 1, 0) x (1, 0, 0)
  line L0 (19.3, 77.3) -> (-13, 77.3) projected
  line L1 (-13, 77.3) -> (-13, 75.3) projected
  line L2 (-13, 75.3) -> (19.3, 75.3) projected
  line L3 (19.3, 75.3) -> (19.3, 77.3) projected
  line L4 (19.3, 100) -> (-13, 100) projected
  line L5 (-13, 100) -> (-13, 98) projected
  line L6 (-13, 98) -> (19.3, 98) projected
  line L7 (19.3, 98) -> (19.3, 100) projected
  line L8 (-16, 98) -> (-16, 93) projected
  line L9 (-16, 93) -> (-17, 93) projected
  line L10 (-17, 81.3) -> (-17, 93) projected
  line L11 (-16, 81.3) -> (-17, 81.3) projected
  line L12 (-16, 81.3) -> (-16, 77.3) projected
  line L13 (-14.5, 77.3) -> (-16, 77.3) projected
  line L14 (-14.5, 77.3) -> (-13, 77.3) projected
  line L15 (-13, 77.3) -> (17.3, 77.3) projected
  line L16 (17.3, 77.3) -> (17.3, 78.3) projected
  line L17 (17.3, 78.3) -> (-15, 78.3) projected
  line L18 (-15, 78.3) -> (-15, 97) projected
  line L19 (-15, 97) -> (17.3, 97) projected
  line L20 (17.3, 97) -> (17.3, 98) projected
  line L21 (17.3, 98) -> (-13, 98) projected
  line L22 (-13, 98) -> (-14.5, 98) projected
  line L23 (-14.5, 98) -> (-16, 98) projected
  line L24 (17.3, 77.3) -> (19.3, 77.3)
  line L25 (19.3, 77.3) -> (19.3, 98)
  line L26 (19.3, 98) -> (17.3, 98)
  line L27 (17.3, 98) -> (17.3, 77.3)
  point P0 (75.2, 54)
  constraints: 8 end point, 2 parallel, 1 horizontal, 1 perpendicular
extrude "Extrusion55" add sketch "Sketch66" along normal blind 3.2 contours L0 L16 L27 L20 L6 L25
sketch "Sketch68" plane through (-88.2, 6.2, -44) normal (0, 0, 1) x (1, 0, 0)
  line L0 (6, 0) -> (12, 0)
  line L1 (12, 0) -> (12, -1)
  line L2 (12, -1) -> (6, -1)
  line L3 (6, -1) -> (6, 0)
  line L4 (20.3, 0) -> (26.3, 0)
  line L5 (26.3, 0) -> (26.3, -1)
  line L6 (26.3, -1) -> (20.3, -1)
  line L7 (20.3, -1) -> (20.3, 0)
  line L8 (0, 0) -> (32.3, 0) projected
  line L9 (0, -2.7) -> (0, 0) projected
  line L10 (32.3, -1) -> (32.3, 0) projected
  point P0 (88.2, -6.2)
  point P1 (9, 0)
  point P2 (23.3, 0)
  dimension "d427" = 6
  dimension "d428" = 1
  dimension "d429" = 1
  dimension "d430" = 6
  dimension "d431" = 6
  dimension "d432" = 6
  constraints: 16 end point, 4 parallel, 2 horizontal, 2 midpoint, 2 perpendicular, 2 point on line
  measures "d427" distance of L1.end L2.end
  measures "d428" distance of L0.end L1.end
  measures "d429" distance of L6.end L4.start
  measures "d430" distance of L5.end L6.end
  measures "d431" distance between parallel lines of L3 L9
  measures "d432" distance between parallel lines of L10 L5
extrude "Extrusion56" add sketch "Sketch68" along normal blind 0.2
chamfer "Chamfer8" distance 1 distance2 0.2 1 edges at (-79.2, 6.2, -43.8) measured on face at (-79.2, 5.7, -43.8)
chamfer "Chamfer9" distance 1 distance2 0.2 1 edges at (-64.9, 6.2, -43.8) measured on face at (-64.9, 5.7, -43.8)
sketch "Sketch69" plane through (-55.9, 6.2, -23.3) normal (0, 0, -1) x (-1, 0, 0)
  line L0 (31.3, -2.2) -> (-2.7, -2.2) projected
  line L1 (12, 0) -> (12, -1) projected
  line L2 (12, -1) -> (6, -1) projected
  line L3 (6, -1) -> (6, 0) projected
  line L4 (6, 0) -> (12, 0) projected
  line L5 (26.3, 0) -> (26.3, -1) projected
  line L6 (26.3, -1) -> (20.3, -1) projected
  line L7 (20.3, -1) -> (20.3, 0) projected
  line L8 (20.3, 0) -> (26.3, 0) projected
  line L9 (6, -1) -> (12, -1)
  line L10 (12, -1) -> (12, 0)
  line L11 (12, 0) -> (6, 0)
  line L12 (6, 0) -> (6, -1)
  line L13 (20.3, -1) -> (26.3, -1)
  line L14 (26.3, -1) -> (26.3, 0)
  line L15 (26.3, 0) -> (20.3, 0)
  line L16 (20.3, 0) -> (20.3, -1)
  point P0 (-55.9, -6.2)
  constraints: 16 end point, 4 parallel, 2 horizontal, 2 perpendicular
extrude "Extrusion57" add sketch "Sketch69" along normal blind 0.2
chamfer "Chamfer10" distance 1 distance2 0.2 1 edges at (-64.9, 6.2, -23.5) measured on face at (-64.9, 5.7, -23.5)
chamfer "Chamfer11" distance 1 distance2 0.2 1 edges at (-79.2, 6.2, -23.5) measured on face at (-79.2, 5.7, -23.5)
sketch "Sketch71" plane through (92.2, 0, 57) normal (1, 0, 0) x (0, 0, -1)
  line L0 (35.95, 2) -> (35.95, 16) projected
  line L1 (23.5, 1) -> (10, 1) projected
  line L2 (14.45, 13.5) -> (33.45, 13.5)
  line L3 (33.45, 13.5) -> (33.45, 2)
  line L4 (33.45, 2) -> (14.45, 2)
  line L5 (14.45, 2) -> (14.45, 13.5)
  line L6 (16.35, 12.5) -> (26.35, 12.5)
  line L7 (26.35, 12.5) -> (26.35, 3)
  line L8 (26.35, 3) -> (16.35, 3)
  line L9 (16.35, 3) -> (16.35, 12.5)
  circle A0 centre (30.45, 7.75) radius 1.25
  line L10 (33.45, 7.75) -> (14.45, 7.75) construction
  line L11 (0, 0) -> (114, 0) projected
  point P0 (57, 0)
  point P1 (26.35, 7.75)
  dimension "d449" = 2.5
  dimension "d450" = 19
  dimension "d451" = 11.5
  dimension "d452" = 2.5
  dimension "d453" = 9.5
  dimension "d454" = 10
  dimension "d455" = 1.9
  dimension "d456" = 16
  dimension "d465" = 2
  constraints: 18 end point, 4 parallel, 3 midpoint, 2 horizontal, 2 perpendicular, 2 point on line, 1 centre point
  measures "d449" distance between parallel lines of L0 L3
  measures "d450" distance of L2.start L2.end
  measures "d451" distance of L2.end L3.end
  measures "d452" diameter of A0
  measures "d453" distance of L6.end L7.end
  measures "d454" distance of L7.end L8.end
  measures "d455" distance between parallel lines of L9 L5
  measures "d456" distance from line of L5 A0.centre
  measures "d465" distance between parallel lines of L4 L11
extrude "Extrusion58" cut sketch "Sketch71" against normal up to surface (2 mm away) contours L6 L7 L8 L9 | A0